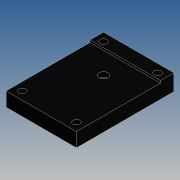
# Autodesk Inventor part: P101
Saved by Autodesk Inventor 2019 (Build 230136000, 136)
## iProperties
Created: 2016-06-02
Part Number: P101
Material: Aluminium
Document SubType Name: Modeling
Designer: serge.amoos
Density: 2.7 g/cm^3
Appearance: Smooth - Black
Description: Plaque de base
Author: serge.amoos
Autodesk Inventor part; units mm, degrees
ref_plane "YZ Plane" through (0, 0, 0) normal (1, 0, 0) x (0, 1, 0)
ref_plane "XZ Plane" through (0, 0, 0) normal (0, 1, 0) x (-1, 0, 0)
ref_plane "XY Plane" through (0, 0, 0) normal (0, 0, 1) x (1, 0, 0)
sketch "Sketch1" plane through (0, 0, 0) normal (0, 0, 1) x (1, 0, 0)
  line L0 (-45.5, 0) -> (45.5, 0) construction
  line L1 (0, -75.5) -> (0, 50.5) construction
  line L2 (-32.5, 32.5) -> (32.5, 32.5)
  line L3 (32.5, 32.5) -> (32.5, -57.5)
  line L4 (32.5, -57.5) -> (-32.5, -57.5)
  line L5 (-32.5, -57.5) -> (-32.5, 32.5)
  point P0 (0, 0)
  point P1 (0, 32.5)
  point P2 (32.5, -12.5)
  dimension "d0" = 65
  dimension "d28" = 32.5
  dimension "d29" = 57.5
  constraints: 8 end point, 2 midpoint, 2 parallel, 1 horizontal, 1 perpendicular, 1 point on line
  measures "d0" distance of L2.start L2.end
  measures "d28" distance between parallel lines of L0 L2
  measures "d29" distance between parallel lines of L4 L0
extrude "Extrusion1" add sketch "Sketch1" along normal blind 15
sketch "Sketch2" plane through (0, 0, 0) normal (0, 0, -1) x (-1, 0, 0)
  point P0 (0, 0)
hole "Hole1" at (0, 0, 0) direction (0, 0, 1) diameter 8.2 end through all counterbore diameter 15 counterbore depth 8.5
sketch "Sketch3" plane through (0, 0, 15) normal (0, 0, 1) x (1, 0, 0)
  line L0 (-45.5, 0) -> (45.5, 0) projected
  line L1 (0, -75.5) -> (0, 50.5) projected
  point P0 (0, 0)
  point P1 (-25, 25)
  dimension "d16" = 25
  dimension "d17" = 25
  measures "d16" distance from line of L1 point (-25, 25)
  measures "d17" distance from line of L0 point (-25, 25)
hole "Hole2" at (-25, 25, 15) direction (0, 0, -1) diameter 6.3 end through all
pattern_linear "Rectangular Pattern2" count 2 spacing 50 along (1, 0, 0) count 2 spacing 75 along (0, -1, 0) of "Hole2"
sketch "Sketch4" plane through (0, 0, 15) normal (0, 0, 1) x (1, 0, 0)
  circle A0 centre (0, 0) radius 4.1 construction
  line L0 (32.5, 32.5) -> (32.5, -57.5) construction
  line L1 (32.5, -57.5) -> (-32.5, -57.5) construction
  line L2 (-32.5, -57.5) -> (-32.5, 32.5) construction
  line L3 (-32.5, 32.5) -> (32.5, 32.5) construction
  line L4 (-32.5, -57.5) -> (32.5, -57.5)
  line L5 (32.5, -57.5) -> (32.5, 20)
  line L6 (32.5, 20) -> (-32.5, 20)
  line L7 (-32.5, 20) -> (-32.5, -57.5)
  circle A1 centre (25, -50) radius 3.15 projected
  circle A2 centre (-25, -50) radius 3.15 projected
  circle A3 centre (25, 25) radius 3.15 projected
  circle A4 centre (-25, 25) radius 3.15 projected
  dimension "d42" = 20
  constraints: 8 end point, 2 parallel, 1 horizontal, 1 perpendicular, 1 point on line
  measures "d42" distance from line of point (0, 0) L6
extrude "Extrusion2" cut sketch "Sketch4" against normal blind 2 contours L7 L6 L5 L4 | A1 | A2
equation "\"d17\" = d16"
body "Solid1"
